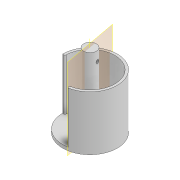
# Autodesk Inventor part: Hand Holder
Saved by Autodesk Inventor 2020 (Build 240168000, 168)
## iProperties
Created: 2019-12-04
Part Number: Hand Holder
Material: Generic
Document SubType Name: Modeling
Designer: ball
Density: 1 g/cm^3
Appearance: Default
Author: ball
Autodesk Inventor part; units mm, degrees
ref_plane "YZ Plane" through (0, 0, 0) normal (1, 0, 0) x (0, 1, 0)
ref_plane "XZ Plane" through (0, 0, 0) normal (0, 1, 0) x (-1, 0, 0)
ref_plane "XY Plane" through (0, 0, 0) normal (0, 0, 1) x (1, 0, 0)
sketch "Sketch1" plane through (0, 0, 0) normal (0, 1, 0) x (-1, 0, 0)
  circle A0 centre (0, 0) radius 53.975
  dimension "d0" = 107.95
  constraints: 1 centre point, 1 coincident
  measures "d0" diameter of A0
extrude "Extrusion1" add sketch "Sketch1" along normal blind 107.95
sketch "Sketch2" plane through (0, 107.95, 0) normal (0, 1, 0) x (1, 0, 0)
  arc A0 (-1.614, -49.186) -> (-49.186, -1.614) centre (0, 0) ccw
  circle A1 centre (0, 0) radius 53.975 projected
  line L0 (9.8864, -53.0619) -> (14.2923, -39.9886)
  line L1 (14.2923, -39.9886) -> (-59.1143, -15.2492)
  line L2 (-59.1143, -15.2492) -> (-53.975, 0)
  line L3 (-53.975, 0) -> (-49.186, -1.614)
  line L4 (-1.614, -49.186) -> (9.8864, -53.0619)
  dimension "d3" = 98.425
  constraints: 10 end point, 4 point on circle, 3 parallel, 2 perpendicular, 1 centre point, 1 coincident
  measures "d3" diameter of A0
extrude "Extrusion2" cut sketch "Sketch2" against normal blind 101.6 contours L4 A1 L1 L0 A0 | L0 L1 A1 L3 A0
sketch "Sketch3" plane through (0, 6.35, 0) normal (0, 1, 0) x (1, 0, 0)
  circle A0 centre (0, 0) radius 12.7
  dimension "d7" = 25.4
  constraints: 1 centre point, 1 coincident
  measures "d7" diameter of A0
extrude "Extrusion3" add sketch "Sketch3" along normal blind 139.7
ref_plane "Work Plane1" through (0, 6.35, 0) normal (0.9831, 0, -0.1832) x (0, 1, 0)
sketch "Sketch4" plane through (0, 6.35, 0) normal (0.9831, 0, -0.1832) x (0, 1, 0)
  circle A0 centre (120.65, 0) radius 3.175
  line L0 (139.7, -12.7) -> (139.7, 12.7) projected
  point P0 (-6.35, 0)
  dimension "d10" = 6.35
  dimension "d11" = 19.05
  constraints: 1 centre point
  measures "d10" diameter of A0
  measures "d11" distance from line of L0 A0.centre
extrude "Extrusion4" cut sketch "Sketch4" along normal through all
sketch "Sketch5" plane through (0, 6.35, 0) normal (0.9831, 0, -0.1832) x (0, 1, 0)
  circle A0 centre (120.65, 0) radius 3.175 projected
  circle A1 centre (120.65, 0) radius 3.175
  point P0 (-6.35, 0)
  constraints: 1 centre point, 1 coincident
extrude "Extrusion5" cut sketch "Sketch5" against normal blind 139.7
fillet "Fillet2" radius 2.54 2 edges at (-49.186, 57.15, 1.614) (-1.614, 57.15, 49.186)
body "Solid1"
